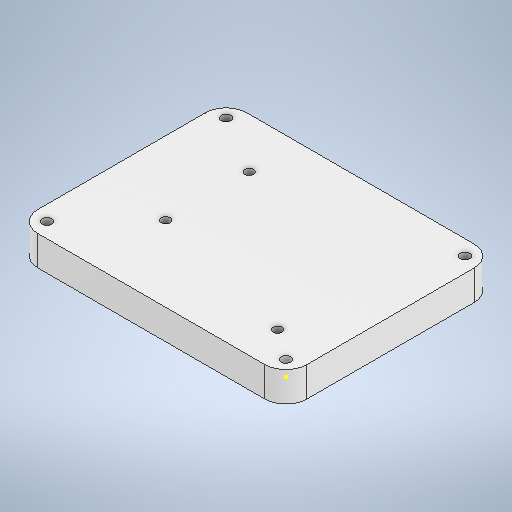
# Autodesk Inventor part: Módulo de fixação Arduíno
Saved by Autodesk Inventor 2025 (Build 290162000, 162)
## iProperties
Created: 2024-04-25
Part Number: Módulo de fixação Arduíno
Material: PPS Plastic
Document SubType Name: Modeling
Designer: kaike
Density: 1.637 g/cm^3
Appearance: Smooth - White
Mass: 102.016 g
Surface Area: 159.193 cm^2
Volume: 62.3189 cm^3
Author: kaike
Autodesk Inventor part; units mm, degrees
ref_plane "YZ Plane" through (0, 0, 0) normal (1, 0, 0) x (0, 1, 0)
ref_plane "XZ Plane" through (0, 0, 0) normal (0, 1, 0) x (-1, 0, 0)
ref_plane "XY Plane" through (0, 0, 0) normal (0, 0, 1) x (1, 0, 0)
sketch "Sketch1" plane through (0, 0, 0) normal (0, 1, 0) x (-1, 0, 0)
  line L0 (0, 0) -> (0, -70)
  line L1 (0, -70) -> (90, -70)
  line L2 (90, -70) -> (90, 0)
  line L3 (90, 0) -> (0, 0)
  circle A0 centre (85, -65) radius 1.6095
  circle A1 centre (85, -5) radius 1.6095
  circle A2 centre (85, -5) radius 1.6095
  circle A3 centre (85, -65) radius 1.6095
  circle A4 centre (5, -65) radius 1.6095
  circle A5 centre (5, -5) radius 1.6095
  circle A6 centre (5, -65) radius 1.6095
  circle A7 centre (5, -5) radius 1.6095
  dimension "d0" = 70
  dimension "d1" = 90
  dimension "d5" = 5
  dimension "d6" = 3.2191
  constraints: 8 centre point, 8 end point, 2 perpendicular, 1 parallel, 1 vertical
  measures "d0" distance of L0.start L0.end
  measures "d1" distance of L0.end L1.end
  measures "d5" distance from line of L2 A0.centre
  measures "d6" diameter of A2
extrude "Extrusion1" add sketch "Sketch1" along normal blind 15
sketch "Sketch2" plane through (0, 15, 0) normal (0, 1, 0) x (1, 0, 0)
  line L0 (-90, 70) -> (-90, 0) projected
  line L1 (-90, 0) -> (0, 0) projected
  line L2 (-90, 0) -> (0, 0)
  line L3 (0, 70) -> (-90, 70) projected
  line L4 (0, 0) -> (0, 70)
  line L5 (0, 70) -> (-90, 70)
  line L6 (-90, 70) -> (-90, 0)
  constraints: 8 end point, 2 collinear, 2 perpendicular
extrude "Extrusion2" cut sketch "Sketch2" against normal blind 5
fillet "Fillet1" radius 7 4 edges at (-90, 5, -70) (-90, 5, 0) (0, 5, -70) (0, 5, 0)
sketch "Sketch3" plane through (0, 0, 0) normal (0, -1, 0) x (1, 0, 0)
  circle A0 centre (-85, -65) radius 1.6095 projected
  circle A1 centre (-85, -65) radius 1.6095
  circle A2 centre (-85, -5) radius 1.6095 projected
  circle A3 centre (-85, -5) radius 1.6095
  circle A4 centre (-5, -5) radius 1.6095 projected
  circle A5 centre (-5, -5) radius 1.6095
  circle A6 centre (-5, -65) radius 1.6095 projected
  circle A7 centre (-5, -65) radius 1.6095
  point P0 (0, 0)
  constraints: 4 centre point, 4 coincident
extrude "Extrusion3" add sketch "Sketch3" against normal blind 2
sketch "Sketch4" plane through (0, 10, 0) normal (0, 1, 0) x (1, 0, 0)
  point P0 (0, 0)
sketch "Sketch5" plane through (0, 10, 0) normal (0, 1, 0) x (1, 0, 0)
  circle A0 centre (-15, 12.25) radius 1.5
  circle A1 centre (-65.5, 53.25) radius 1.5
  circle A2 centre (-65.5, 25.25) radius 1.5
  point P0 (0, 0)
  constraints: 3 centre point
extrude "Extrusion4" cut sketch "Sketch5" against normal blind 7
